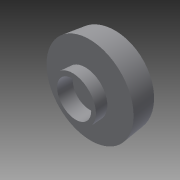
# Autodesk Inventor part: Lens
Saved by Autodesk Inventor 2015 SP1 (Build 190203100, 203)
## iProperties
Created: 2015-05-04
Part Number: Lens
Material: Generic
Document SubType Name: Modeling
Designer: Brandon
Density: 1 g/cm^3
Appearance: Default
Author: Brandon
Autodesk Inventor part; units mm, degrees
ref_plane "YZ Plane" through (0, 0, 0) normal (1, 0, 0) x (0, 1, 0)
ref_plane "XZ Plane" through (0, 0, 0) normal (0, 1, 0) x (-1, 0, 0)
ref_plane "XY Plane" through (0, 0, 0) normal (0, 0, 1) x (1, 0, 0)
sketch "Sketch1" plane through (0, 0, 0) normal (0, 0, 1) x (1, 0, 0)
  line L0 (-49.8, -32.05) -> (49.8, -32.05) projected
  line L1 (49.8, 32.05) -> (-49.8, 32.05) projected
  circle A0 centre (0, 0) radius 25.4
  line L2 (49.8, -32.05) -> (49.8, 32.05) projected
  line L3 (-49.8, 32.05) -> (-49.8, -32.05) projected
  dimension "d0" = 50.8
  constraints: 1 centre point, 1 coincident
  measures "d0" diameter of A0
extrude "Extrusion1" add sketch "Sketch1" along normal blind 12.7 contours A0
sketch "Sketch2" plane through (0, 0, 12.7) normal (0, 0, 1) x (1, 0, 0)
  circle A0 centre (0, 0) radius 25.4 projected
  circle A1 centre (0, 0) radius 12.7
  dimension "d3" = 25.4
  constraints: 1 centre point, 1 coincident
  measures "d3" diameter of A1
extrude "Extrusion2" add sketch "Sketch2" along normal blind 6.35 contours A1
shell "Shell1" thickness 2.54 removed faces 1 at (-3.6254, -0.9542, 19.05)
sketch "Sketch3" plane through (0, 0, 2.54) normal (0, 0, 1) x (1, 0, 0)
  line L0 (-4.445, -3.175) -> (4.445, -3.175)
  line L1 (4.445, -3.175) -> (4.445, 3.175)
  line L2 (4.445, 3.175) -> (-4.445, 3.175)
  line L3 (-4.445, 3.175) -> (-4.445, -3.175)
  line L4 (-4.445, -3.175) -> (4.445, 3.175) construction
  line L5 (4.445, -3.175) -> (-4.445, 3.175) construction
  point P0 (0, 0)
  dimension "d7" = 8.89
  dimension "d8" = 6.35
  constraints: 12 end point, 2 midpoint, 2 parallel, 1 horizontal, 1 perpendicular
  measures "d7" distance of L1.end L2.end
  measures "d8" distance of L2.end L0.start
extrude "Extrusion3" cut sketch "Sketch3" against normal blind 1
sketch "Sketch4" plane through (0, 0, 1.54) normal (0, 0, 1) x (1, 0, 0)
  line L0 (4.445, -3.175) -> (-4.445, -3.175) projected
  line L1 (4.445, 3.175) -> (4.445, -3.175) projected
  line L2 (-4.445, 3.175) -> (4.445, 3.175) projected
  line L3 (-4.445, -3.175) -> (-4.445, 3.175) projected
  line L4 (-4.445, -3.175) -> (-4.445, 3.175) projected
  line L5 (4.445, -0.125) -> (-4.445, -0.125)
  line L6 (-4.445, -0.125) -> (-4.445, 0.125)
  line L7 (-4.445, 0.125) -> (4.445, 0.125)
  line L8 (4.445, 0.125) -> (4.445, -0.125)
  line L9 (4.445, -0.125) -> (-4.445, 0.125) construction
  line L10 (-4.445, -0.125) -> (4.445, 0.125) construction
  point P0 (0, 0)
  dimension "d11" = 0.25
  constraints: 12 end point, 2 midpoint, 2 parallel, 1 horizontal, 1 perpendicular, 1 point on line
  measures "d11" distance of L5.end L6.end
extrude "Extrusion4" cut sketch "Sketch4" against normal blind 1 contours L5 L3 L7 L1
body "Solid1"
